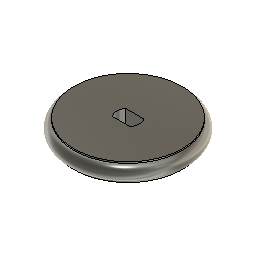
CAR-WHEEL (Autodesk Fusion 360 design; units mm, degrees)
Autodesk Fusion 360 part; units mm, degrees
sketch "Sketch1" plane through (0, 0, 0) normal (0, 0, 1) x (1, 0, 0)
  circle A0 centre (0, 0) radius 12
  circle A1 centre (0, 0) radius 2.5
  circle A2 centre (0, 0) radius 4.5
  line L0 (-2, 1.5) -> (2, 1.5)
  line L1 (-2, -1.5) -> (2, -1.5)
  dimension "d2" = 24
  dimension "d3" = 5
  dimension "d4" = 9
  dimension "d5" = 1.5
  dimension "d6" = 1.5
  constraint coincident A0.centre A1.centre
  constraint concentric A1 A2
  constraint coincident A1 L0.start
  constraint coincident A1 L0.end
  constraint horizontal L0
  constraint coincident A1 L1.start
  constraint coincident A1 L1.end
  constraint parallel L0 L1
  measures "d2" diameter of A0
  measures "d3" diameter of A1
  measures "d4" diameter of A2
  measures "d5" vertical distance of A0.centre L0.end
  measures "d6" vertical distance of A0.centre L1.end
extrude "Extrude5" add sketch "Sketch1" along normal mid plane 4 contours A0 | A1 L0 | A1 L1 | A2 makes body 1
torus "TorusPrimitive1" cut centre line diameter 23 section diameter 3.5 placed x (1, 0, 0) y (0, 1, 0) z (0, 0, 1) at (0, 0, 0) bodies 1
torus "TorusPrimitive1'" add centre line diameter 23 section diameter 3.5 placed x (1, 0, 0) y (0, 1, 0) z (0, 0, 1) at (0, 0, 0) separate body makes body 2 in component "Oring"
extrude "Extrude2" [suppressed]
extrude "Extrude1" [suppressed]
extrude "Extrude3" [suppressed]
extrude "Extrude4" [suppressed]
component "Oring" placed x (1, 0, 0) y (0, 1, 0) z (0, 0, 1) at (0, 0, 0)
named bodies: "Wheels-Body"
